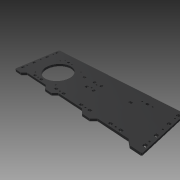
# Autodesk Inventor part: back
Saved by Autodesk Inventor 2014 (Build 180170000, 170)
## iProperties
Created: 2013-12-05
Part Number: back
Material: Plywood, Finish
Document SubType Name: Modeling
Designer: buben
Density: 0.552 g/cm^3
Appearance: Plywood - New
Author: buben
Subject: Laser Cutted
Autodesk Inventor part; units mm, degrees
ref_plane "YZ Plane" through (0, 0, 0) normal (1, 0, 0) x (0, 1, 0)
ref_plane "XZ Plane" through (0, 0, 0) normal (0, 1, 0) x (-1, 0, 0)
ref_plane "XY Plane" through (0, 0, 0) normal (0, 0, 1) x (1, 0, 0)
sketch "Sketch1" plane through (0, 0, 0) normal (0, 0, 1) x (1, 0, 0)
  line L0 (0, 0) -> (355, 0)
  line L1 (355, 0) -> (355, 120.5)
  line L2 (355, 120.5) -> (0, 120.5)
  line L3 (0, 120.5) -> (0, 0)
  dimension "d0" = 120.5
  dimension "d1" = 355
  constraints: 8 end point, 2 parallel, 1 horizontal, 1 perpendicular
  measures "d0" distance of L2.end L0.start
  measures "d1" distance of L0.start L0.end
extrude "Extrusion1" add sketch "Sketch1" along normal blind 6.5
sketch "Sketch3" plane through (0, 0, 6.5) normal (0, 0, 1) x (1, 0, 0)
  line L0 (0, 0) -> (355, 0) projected
  line L1 (355, 120.5) -> (0, 120.5) projected
  line L2 (0, 120.5) -> (0, 0) projected
  circle A0 centre (64.5, 96) radius 4
  circle A1 centre (290.5, 96) radius 4
  line L3 (64.5, 96) -> (290.5, 96) construction
  point P0 (177.5, 96)
  point P1 (177.5, 120.5)
  dimension "d9" = 8
  dimension "d10" = 96
  dimension "d11" = 226
  constraints: 2 centre point, 2 end point, 2 midpoint, 1 equal radius, 1 horizontal alignment, 1 perpendicular, 1 vertical alignment
  measures "d9" diameter of A0
  measures "d10" distance from line of L0 L3.start
  measures "d11" distance of L3.start L3.end
extrude "Extrusion3" cut sketch "Sketch3" against normal through all
sketch "Sketch4" plane through (0, 0, 6.5) normal (0, 0, 1) x (1, 0, 0)
  line L0 (0, 0) -> (355, 0) projected
  line L1 (355, 120.5) -> (0, 120.5) projected
  line L2 (0, 120.5) -> (0, 0) projected
  circle A0 centre (6.25, 18.5) radius 2.25
  circle A1 centre (6.25, 57.5) radius 2.25
  circle A2 centre (6.25, 96.5) radius 2.25
  line L3 (177.5, 120.5) -> (177.5, 0) construction
  line L4 (3, 112) -> (9.5, 112)
  line L5 (9.5, 112) -> (9.5, 104)
  line L6 (9.5, 104) -> (3, 104)
  line L7 (3, 104) -> (3, 112)
  line L8 (3, 81) -> (9.5, 81)
  line L9 (9.5, 81) -> (9.5, 73)
  line L10 (9.5, 73) -> (3, 73)
  line L11 (3, 73) -> (3, 81)
  line L12 (3, 42) -> (9.5, 42)
  line L13 (9.5, 42) -> (9.5, 34)
  line L14 (9.5, 34) -> (3, 34)
  line L15 (3, 34) -> (3, 42)
  line L16 (3, 11) -> (9.5, 11)
  line L17 (9.5, 11) -> (9.5, 3)
  line L18 (9.5, 3) -> (3, 3)
  line L19 (3, 3) -> (3, 11)
  line L20 (6.25, 18.5) -> (6.25, 57.5) construction
  line L21 (6.25, 57.5) -> (6.25, 96.5) construction
  circle A3 centre (348.75, 18.5) radius 2.25
  circle A4 centre (348.75, 57.5) radius 2.25
  circle A5 centre (348.75, 96.5) radius 2.25
  line L22 (352, 112) -> (345.5, 112)
  line L23 (345.5, 112) -> (345.5, 104)
  line L24 (345.5, 104) -> (352, 104)
  line L25 (352, 104) -> (352, 112)
  line L26 (352, 81) -> (345.5, 81)
  line L27 (345.5, 81) -> (345.5, 73)
  line L28 (345.5, 73) -> (352, 73)
  line L29 (352, 73) -> (352, 81)
  line L30 (352, 42) -> (345.5, 42)
  line L31 (345.5, 42) -> (345.5, 34)
  line L32 (345.5, 34) -> (352, 34)
  line L33 (352, 34) -> (352, 42)
  line L34 (352, 11) -> (345.5, 11)
  line L35 (345.5, 11) -> (345.5, 3)
  line L36 (345.5, 3) -> (352, 3)
  line L37 (352, 3) -> (352, 11)
  line L38 (348.75, 18.5) -> (348.75, 57.5) construction
  line L39 (348.75, 57.5) -> (348.75, 96.5) construction
  point P0 (6.25, 104)
  point P1 (3, 38)
  point P2 (6.25, 38)
  point P3 (3, 77)
  point P4 (6.25, 77)
  point P5 (348.75, 104)
  point P6 (352, 38)
  point P7 (348.75, 38)
  point P8 (352, 77)
  point P9 (348.75, 77)
  dimension "d14" = 18.5
  dimension "d15" = 39
  dimension "d16" = 39
  dimension "d17" = 4.5
  dimension "d18" = 6.5
  dimension "d19" = 8
  dimension "d20" = 8
  dimension "d21" = 8
  dimension "d22" = 8
  dimension "d23" = 3
  dimension "d27" = 23
  dimension "d28" = 3
  constraints: 74 end point, 24 symmetric about line, 9 parallel, 7 collinear, 7 midpoint, 6 centre point, 4 horizontal, 4 perpendicular, 3 vertical alignment, 2 equal radius, 2 horizontal alignment, 3 other
  measures "d14" distance from line of L0 L20.start
  measures "d15" distance of L20.start L20.end
  measures "d16" distance of L20.end L21.end
  measures "d17" diameter of A0
  measures "d18" distance of L4.start L4.end
  measures "d19" distance of L6.end L4.start
  measures "d20" distance of L10.end L8.start
  measures "d21" distance of L14.end L12.start
  measures "d22" distance of L18.end L16.start
  measures "d23" distance between parallel lines of L0 L18
  measures "d27" distance between parallel lines of L8 L6
  measures "d28" distance between parallel lines of L2 L7
extrude "Extrusion4" cut sketch "Sketch4" against normal through all
sketch "Sketch5" plane through (0, 0, 6.5) normal (0, 0, 1) x (1, 0, 0)
  line L0 (0, 0) -> (355, 0) projected
  line L1 (51, 9.5) -> (59, 9.5)
  line L2 (59, 9.5) -> (59, 3)
  line L3 (59, 3) -> (51, 3)
  line L4 (51, 3) -> (51, 9.5)
  line L5 (74, 9.5) -> (82, 9.5)
  line L6 (82, 9.5) -> (82, 3)
  line L7 (82, 3) -> (74, 3)
  line L8 (74, 3) -> (74, 9.5)
  line L9 (59, 9.5) -> (74, 3) construction
  line L10 (74, 9.5) -> (59, 3) construction
  circle A0 centre (66.5, 6.25) radius 2.25
  line L11 (125, 9.5) -> (133, 9.5)
  line L12 (133, 9.5) -> (133, 3)
  line L13 (133, 3) -> (125, 3)
  line L14 (125, 3) -> (125, 9.5)
  line L15 (148, 9.5) -> (156, 9.5)
  line L16 (156, 9.5) -> (156, 3)
  line L17 (156, 3) -> (148, 3)
  line L18 (148, 3) -> (148, 9.5)
  line L19 (133, 9.5) -> (148, 3) construction
  line L20 (148, 9.5) -> (133, 3) construction
  circle A1 centre (140.5, 6.25) radius 2.25
  line L21 (199, 9.5) -> (207, 9.5)
  line L22 (207, 9.5) -> (207, 3)
  line L23 (207, 3) -> (199, 3)
  line L24 (199, 3) -> (199, 9.5)
  line L25 (222, 9.5) -> (230, 9.5)
  line L26 (230, 9.5) -> (230, 3)
  line L27 (230, 3) -> (222, 3)
  line L28 (222, 3) -> (222, 9.5)
  line L29 (207, 9.5) -> (222, 3) construction
  line L30 (222, 9.5) -> (207, 3) construction
  circle A2 centre (214.5, 6.25) radius 2.25
  line L31 (273, 9.5) -> (281, 9.5)
  line L32 (281, 9.5) -> (281, 3)
  line L33 (281, 3) -> (273, 3)
  line L34 (273, 3) -> (273, 9.5)
  line L35 (296, 9.5) -> (304, 9.5)
  line L36 (304, 9.5) -> (304, 3)
  line L37 (304, 3) -> (296, 3)
  line L38 (296, 3) -> (296, 9.5)
  line L39 (281, 9.5) -> (296, 3) construction
  line L40 (296, 9.5) -> (281, 3) construction
  circle A3 centre (288.5, 6.25) radius 2.25
  line L41 (82, 6.25) -> (125, 6.25) construction
  line L42 (156, 6.25) -> (199, 6.25) construction
  line L43 (230, 6.25) -> (273, 6.25) construction
  line L44 (9.5, 11) -> (9.5, 3) projected
  line L45 (345.5, 3) -> (345.5, 11) projected
  point P0 (288.5, 6.25)
  dimension "d31" = 8
  dimension "d32" = 6.5
  dimension "d33" = 8
  dimension "d34" = 15
  dimension "d35" = 4.5
  dimension "d36" = 8
  dimension "d37" = 6.5
  dimension "d38" = 8
  dimension "d39" = 15
  dimension "d40" = 4.5
  dimension "d41" = 8
  dimension "d42" = 6.5
  dimension "d43" = 8
  dimension "d44" = 15
  dimension "d45" = 4.5
  dimension "d46" = 8
  dimension "d47" = 6.5
  dimension "d48" = 8
  dimension "d49" = 15
  dimension "d50" = 4.5
  dimension "d51" = 3
  dimension "d88" = 57
  dimension "d89" = 57
  constraints: 86 end point, 16 parallel, 11 midpoint, 10 collinear, 8 horizontal, 8 perpendicular, 4 centre point, 3 horizontal alignment
  measures "d31" distance of L1.start L1.end
  measures "d32" distance of L3.end L1.start
  measures "d33" distance of L5.start L5.end
  measures "d34" distance between parallel lines of L8 L2
  measures "d35" diameter of A0
  measures "d36" distance of L14.end L11.end
  measures "d37" distance of L14.start L14.end
  measures "d38" distance of L20.start L15.end
  measures "d39" distance between parallel lines of L18 L12
  measures "d40" diameter of A1
  measures "d41" distance of L24.end L21.end
  measures "d42" distance of L24.start L24.end
  measures "d43" distance of L30.start L25.end
  measures "d44" distance between parallel lines of L28 L22
  measures "d45" diameter of A2
  measures "d46" distance of L34.end L31.end
  measures "d47" distance of L34.start L34.end
  measures "d48" distance of L40.start L35.end
  measures "d49" distance between parallel lines of L38 L32
  measures "d50" diameter of A3
  measures "d51" distance between parallel lines of L0 L3
  measures "d88" distance from line of L44 A0.centre
  measures "d89" distance from line of L45 point (288.5, 6.25)
extrude "Extrusion5" cut sketch "Sketch5" against normal through all
sketch "Sketch6" plane through (0, 0, 6.5) normal (0, 0, 1) x (1, 0, 0)
  line L0 (0, 0) -> (355, 0) projected
  line L1 (0, 120.5) -> (0, 0) projected
  line L2 (0, 0) -> (0, -10)
  line L3 (0, -10) -> (23, -10)
  line L4 (23, -10) -> (33, 0)
  line L5 (102.6667, 0) -> (112.6667, -10)
  line L6 (112.6667, -10) -> (132.6667, -10)
  line L7 (132.6667, -10) -> (142.6667, 0)
  line L8 (212.3333, 0) -> (222.3333, -10)
  line L9 (222.3333, -10) -> (242.3333, -10)
  line L10 (242.3333, -10) -> (252.3333, 0)
  line L11 (355, 0) -> (355, -10)
  line L12 (355, -10) -> (332, -10)
  line L13 (332, -10) -> (322, 0)
  line L14 (23, -10) -> (112.6667, -10) construction
  line L15 (132.6667, -10) -> (222.3333, -10) construction
  line L16 (242.3333, -10) -> (332, -10) construction
  dimension "d54" = 20
  dimension "d55" = 23
  dimension "d56" = 45
  dimension "d57" = 10
  constraints: 30 end point, 13 collinear, 8 perpendicular, 6 point on line
  measures "d54" distance of L5.end L6.end
  measures "d55" distance of L2.end L3.end
  measures "d56" angle of L4 L3
  measures "d57" distance of L0.start L2.end
extrude "Extrusion6" add sketch "Sketch6" against normal blind 6.5
sketch "Sketch7" plane through (0, 0, 6.5) normal (0, 0, 1) x (1, 0, 0)
  line L0 (355, 120.5) -> (0, 120.5) projected
  line L1 (174, 80.41) -> (181, 80.41) construction
  line L2 (181, 80.41) -> (181, 54.41) construction
  line L3 (181, 54.41) -> (174, 54.41) construction
  line L4 (174, 54.41) -> (174, 80.41) construction
  line L5 (184.25, 82.91) -> (190.75, 82.91)
  line L6 (190.75, 82.91) -> (190.75, 74.91)
  line L7 (190.75, 74.91) -> (184.25, 74.91)
  line L8 (184.25, 74.91) -> (184.25, 82.91)
  line L9 (184.25, 59.91) -> (190.75, 59.91)
  line L10 (190.75, 59.91) -> (190.75, 51.91)
  line L11 (190.75, 51.91) -> (184.25, 51.91)
  line L12 (184.25, 51.91) -> (184.25, 59.91)
  line L13 (164.25, 82.91) -> (170.75, 82.91)
  line L14 (170.75, 82.91) -> (170.75, 74.91)
  line L15 (170.75, 74.91) -> (164.25, 74.91)
  line L16 (164.25, 74.91) -> (164.25, 82.91)
  line L17 (164.25, 59.91) -> (170.75, 59.91)
  line L18 (170.75, 59.91) -> (170.75, 51.91)
  line L19 (170.75, 51.91) -> (164.25, 51.91)
  line L20 (164.25, 51.91) -> (164.25, 59.91)
  line L21 (170.75, 74.91) -> (184.25, 59.91) construction
  line L22 (184.25, 74.91) -> (170.75, 59.91) construction
  circle A0 centre (177.5, 74.91) radius 2.25
  circle A1 centre (177.5, 59.91) radius 2.25
  line L23 (177.5, 74.91) -> (177.5, 59.91) construction
  line L24 (125, 9.5) -> (133, 9.5) projected
  line L25 (174.5, 81.79) -> (180.5, 81.79) construction
  line L26 (180.5, 81.79) -> (180.5, 80.41) construction
  line L27 (180.5, 80.41) -> (174.5, 80.41) construction
  line L28 (174.5, 80.41) -> (174.5, 81.79) construction
  point P0 (0, 0)
  point P1 (177.5, 80.41)
  point P2 (177.5, 120.5)
  point P3 (177.5, 67.41)
  point P4 (174, 67.41)
  point P5 (177.5, 67.41)
  point P6 (177.5, 81.79)
  point P7 (174.5, 81.1)
  dimension "d60" = 7
  dimension "d61" = 26
  dimension "d63" = 8
  dimension "d64" = 6.5
  dimension "d65" = 6.5
  dimension "d66" = 8
  dimension "d67" = 13.5
  dimension "d68" = 15
  dimension "d69" = 4.5
  dimension "d70" = 15
  dimension "d100" = 6
  dimension "d101" = 1.38
  dimension "d102" = 71.6
  constraints: 54 end point, 13 parallel, 8 collinear, 8 midpoint, 6 horizontal, 6 perpendicular, 4 vertical alignment, 2 centre point, 1 equal radius, 1 horizontal alignment, 1 point on line
  measures "d60" distance of L1.start L1.end
  measures "d61" distance of L3.end L1.start
  measures "d63" distance of L15.end L13.start
  measures "d64" distance of L13.start L13.end
  measures "d65" distance of L5.start L5.end
  measures "d66" distance of L19.end L17.start
  measures "d67" distance between parallel lines of L8 L14
  measures "d68" distance between parallel lines of L9 L7
  measures "d69" diameter of A0
  measures "d70" distance of L23.start L23.end
  measures "d100" distance of L25.start L25.end
  measures "d101" distance of L27.end L25.start
  measures "d102" distance from line of L24 point (174.5, 81.1)
extrude "Extrusion7" cut sketch "Sketch7" against normal through all
sketch "Sketch8" plane through (0, 0, 6.5) normal (0, 0, 1) x (1, 0, 0)
  line L0 (164.25, 82.91) -> (170.75, 82.91) projected
  circle A0 centre (64.5, 96) radius 4 projected
  circle A1 centre (290.5, 96) radius 4 projected
  line L1 (355, 120.5) -> (0, 120.5) projected
  circle A2 centre (52.5, 96) radius 2.25
  circle A3 centre (76.5, 96) radius 2.25
  circle A4 centre (278.5, 96) radius 2.25
  circle A5 centre (302.5, 96) radius 2.25
  line L2 (52.5, 96) -> (76.5, 96) construction
  line L3 (278.5, 96) -> (302.5, 96) construction
  point P0 (0, 0)
  dimension "d73" = 24
  dimension "d74" = 4.5
  constraints: 4 centre point, 4 end point, 3 equal radius, 2 coincident, 2 collinear, 2 midpoint, 2 parallel
  measures "d73" distance of L2.start L2.end
  measures "d74" diameter of A2
extrude "Extrusion8" cut sketch "Sketch8" against normal through all contours A2 | A3 | A4 | A5
sketch "Sketch9" plane through (0, 0, 6.5) normal (0, 0, 1) x (1, 0, 0)
  line L0 (74, 9.5) -> (82, 9.5) projected
  line L1 (9.5, 42) -> (9.5, 34) projected
  line L2 (44.5, 87) -> (117, 87) construction
  line L3 (117, 87) -> (117, 14.5) construction
  line L4 (117, 14.5) -> (44.5, 14.5) construction
  line L5 (44.5, 14.5) -> (44.5, 87) construction
  circle A0 centre (44.5, 87) radius 2
  circle A1 centre (117, 87) radius 2
  circle A2 centre (117, 14.5) radius 2
  circle A3 centre (44.5, 14.5) radius 2
  line L6 (40.75, 90.75) -> (120.75, 90.75) construction
  line L7 (120.75, 90.75) -> (120.75, 10.75) construction
  line L8 (120.75, 10.75) -> (40.75, 10.75) construction
  line L9 (40.75, 10.75) -> (40.75, 90.75) construction
  point P0 (0, 0)
  point P1 (80.75, 10.75)
  point P2 (80.75, 14.5)
  point P3 (40.75, 50.75)
  point P4 (44.5, 50.75)
  dimension "d77" = 4
  dimension "d78" = 72.5
  dimension "d79" = 5
  dimension "d80" = 80
  dimension "d81" = 35
  constraints: 16 end point, 4 centre point, 4 coincident, 4 midpoint, 4 parallel, 4 perpendicular, 3 equal radius, 2 horizontal, 1 horizontal alignment, 1 vertical alignment
  measures "d77" diameter of A3
  measures "d78" distance of L4.end L2.start
  measures "d79" distance between parallel lines of L0 L4
  measures "d80" distance of L7.end L8.end
  measures "d81" distance between parallel lines of L1 L5
extrude "Extrusion9" cut sketch "Sketch9" against normal through all
sketch "Sketch10" plane through (0, 0, 6.5) normal (0, 0, 1) x (1, 0, 0)
  circle A0 centre (117, 14.5) radius 2 projected
  circle A1 centre (44.5, 87) radius 2 projected
  line L0 (44.5, 87) -> (117, 87) construction
  line L1 (117, 87) -> (117, 14.5) construction
  line L2 (117, 14.5) -> (44.5, 14.5) construction
  line L3 (44.5, 14.5) -> (44.5, 87) construction
  circle A2 centre (80.75, 50.75) radius 37.5
  line L4 (40.75, 98.6417) -> (120.75, 98.6417)
  line L5 (120.75, 98.6417) -> (120.75, 18.6417)
  line L6 (120.75, 18.6417) -> (40.75, 18.6417)
  line L7 (40.75, 18.6417) -> (40.75, 98.6417)
  point P0 (0, 0)
  point P1 (80.75, 87)
  point P2 (44.5, 50.75)
  point P3 (80.75, 98.6417)
  dimension "d84" = 75
  dimension "d87" = 80
  constraints: 16 end point, 4 parallel, 3 midpoint, 3 perpendicular, 2 coincident, 2 horizontal, 2 vertical alignment, 1 centre point, 1 horizontal alignment
  measures "d84" diameter of A2
  measures "d87" distance of L4.start L4.end
extrude "Extrusion10" cut sketch "Sketch10" against normal through all contours A2 L6 | L6 A2
chamfer "Chamfer1" distance 2 angle 45 4 edges at (355, -10, 3.25) (355, 120.5, 3.25) (0, -10, 3.25) (0, 120.5, 3.25)
sketch "Sketch11" plane through (0, 0, 6.5) normal (0, 0, 1) x (1, 0, 0)
  line L0 (51, 9.5) -> (59, 9.5) projected
  line L1 (345.5, 73) -> (345.5, 81) projected
  line L2 (9.5, 81) -> (9.5, 73) projected
  line L3 (134, 81) -> (142, 81)
  line L4 (142, 81) -> (142, 74.5)
  line L5 (142, 74.5) -> (134, 74.5)
  line L6 (134, 74.5) -> (134, 81)
  line L7 (260.5, 81) -> (268.5, 81)
  line L8 (268.5, 81) -> (268.5, 74.5)
  line L9 (268.5, 74.5) -> (260.5, 74.5)
  line L10 (260.5, 74.5) -> (260.5, 81)
  point P0 (0, 0)
  dimension "d93" = 6.5
  dimension "d94" = 8
  dimension "d95" = 65
  dimension "d96" = 124.5
  dimension "d97" = 77
  constraints: 16 end point, 4 parallel, 3 collinear, 2 horizontal, 2 perpendicular
  measures "d93" distance of L5.end L3.start
  measures "d94" distance of L3.start L3.end
  measures "d95" distance between parallel lines of L0 L5
  measures "d96" distance between parallel lines of L2 L6
  measures "d97" distance between parallel lines of L1 L8
extrude "Extrusion11" cut sketch "Sketch11" against normal through all
equation "\"d89\" = d88"
body "Solid1"
